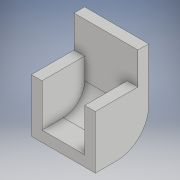
# Autodesk Inventor part: Servo mount
Saved by Autodesk Inventor 2019 (Build 230136000, 136)
## iProperties
Created: 2019-05-30
Part Number: Servo mount
Material: Genérico
Document SubType Name: Modeling
Designer: Daniel Regner
Density: 1 g/cm^3
Appearance: Padrão
Author: Daniel Regner
Autodesk Inventor part; units mm, degrees
ref_plane "YZ Plane" through (0, 0, 0) normal (1, 0, 0) x (0, 1, 0)
ref_plane "XZ Plane" through (0, 0, 0) normal (0, 1, 0) x (-1, 0, 0)
ref_plane "XY Plane" through (0, 0, 0) normal (0, 0, 1) x (1, 0, 0)
sketch "Esboço1" plane through (0, 0, 0) normal (0, 0, 1) x (1, 0, 0)
  line L0 (-12.5, -12.5) -> (-2.5, -12.5)
  line L1 (12.5, 2.5) -> (12.5, 12.5)
  line L2 (12.5, 12.5) -> (-12.5, 12.5)
  line L3 (-12.5, 12.5) -> (-12.5, -12.5)
  line L4 (-12.5, -12.5) -> (12.5, 12.5) construction
  line L5 (12.5, -12.5) -> (-12.5, 12.5) construction
  line L6 (12.5, 12.5) -> (7.5, 12.5)
  line L7 (7.5, 12.5) -> (7.5, 27.5)
  line L8 (7.5, 27.5) -> (12.5, 27.5)
  line L9 (12.5, 27.5) -> (12.5, 12.5)
  arc A0 (-2.5, -12.5) -> (12.5, 2.5) centre (-2.5, 2.5) ccw
  point P0 (0, 0)
  dimension "d0" = 25
  dimension "d1" = 25
  dimension "d2" = 5
  dimension "d3" = 15
  dimension "d4" = 15
  constraints: 20 end point, 4 parallel, 2 horizontal, 2 midpoint, 2 perpendicular, 2 point on circle, 2 point on line, 2 tangent, 1 centre point
  measures "d0" distance of L2.end L1.end
  measures "d1" distance of L1.end L5.start
  measures "d2" distance of L7.end L8.end
  measures "d3" distance of L6.end L7.end
  measures "d4" radius of A0
extrude "Extrusão1" add sketch "Esboço1" along normal blind 30
shell "Casca1" thickness 5 removed faces 2 at (0.8333, 12.5, 10) at (-12.5, 4.1667, 20)
